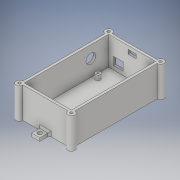
# Autodesk Inventor part: Podstawa
Saved by Autodesk Inventor 2019 (Build 230136000, 136)
## iProperties
Created: 2019-09-16
Part Number: Podstawa
Material: Ogólny
Document SubType Name: Modeling
Designer: mikol
Density: 1 g/cm^3
Appearance: Domyślna
Author: mikol
Autodesk Inventor part; units mm, degrees
ref_plane "YZ Plane" through (0, 0, 0) normal (1, 0, 0) x (0, 1, 0)
ref_plane "XZ Plane" through (0, 0, 0) normal (0, 1, 0) x (-1, 0, 0)
ref_plane "XY Plane" through (0, 0, 0) normal (0, 0, 1) x (1, 0, 0)
sketch "Sketch1" plane through (0, 0, 0) normal (0, 1, 0) x (-1, 0, 0)
  line L0 (32, 55) -> (-32, 55)
  line L1 (-32, 55) -> (-32, -55)
  line L2 (-32, -55) -> (32, -55)
  line L3 (32, -55) -> (32, 55)
  line L4 (32, 55) -> (-32, -55) construction
  line L5 (-32, 55) -> (32, -55) construction
  point P0 (0, 0)
  dimension "d0" = 64
  dimension "d1" = 110
  constraints: 12 end point, 2 midpoint, 2 parallel, 1 horizontal, 1 perpendicular
  measures "d0" distance of L2.end L1.end
  measures "d1" distance of L1.end L0.end
extrude "Extrusion1" add sketch "Sketch1" along normal blind 3
sketch "Sketch2" plane through (0, 3, 0) normal (0, 1, 0) x (1, 0, 0)
  line L0 (-32, -55) -> (32, -55) projected
  line L1 (32, -55) -> (32, 55) projected
  line L2 (32, 55) -> (-32, 55) projected
  line L3 (-32, 55) -> (-32, -55) projected
  line L4 (-32, -55) -> (32, -55)
  line L5 (32, -55) -> (32, 55)
  line L6 (32, 55) -> (-32, 55)
  line L7 (-32, 55) -> (-32, -55)
  line L8 (-32, -55) -> (32, 55) construction
  line L9 (32, -55) -> (-32, 55) construction
  line L10 (-29, -52) -> (29, -52)
  line L11 (29, -52) -> (29, 52)
  line L12 (29, 52) -> (-29, 52)
  line L13 (-29, 52) -> (-29, -52)
  point P0 (0, 0)
  dimension "d4" = 3
  dimension "d5" = 3
  dimension "d6" = 3
  dimension "d7" = 3
  constraints: 20 end point, 4 parallel, 2 horizontal, 2 midpoint, 2 perpendicular
  measures "d4" distance between parallel lines of L2 L12
  measures "d5" distance between parallel lines of L7 L13
  measures "d6" distance between parallel lines of L0 L10
  measures "d7" distance between parallel lines of L1 L11
extrude "Extrusion2" add sketch "Sketch2" along normal blind 35
sketch "Sketch3" plane through (0, 3, 0) normal (0, 1, 0) x (1, 0, 0)
  line L0 (-23.08, -46) -> (23.08, -46)
  line L1 (23.08, -46) -> (23.08, 46)
  line L2 (23.08, 46) -> (-23.08, 46)
  line L3 (-23.08, 46) -> (-23.08, -46)
  circle A0 centre (-23.08, -46) radius 1.25
  circle A1 centre (23.08, -46) radius 1.25
  circle A2 centre (23.08, 46) radius 1.25
  circle A3 centre (-23.08, 33) radius 1.25
  line L4 (-29, -52) -> (-29, 52) projected
  line L5 (29, 52) -> (29, -52) projected
  line L6 (-29, 52) -> (29, 52) projected
  line L7 (29, -52) -> (-29, -52) projected
  circle A4 centre (-23.08, -46) radius 3
  circle A5 centre (-23.08, 33) radius 3
  circle A6 centre (23.08, -46) radius 3
  circle A7 centre (23.08, 46) radius 3
  point P0 (0, 0)
  dimension "d15" = 46.16
  dimension "d16" = 92
  dimension "d17" = 2.5
  dimension "d18" = 2.5
  dimension "d19" = 2.5
  dimension "d20" = 2.5
  dimension "d21" = 79
  dimension "d22" = 5.92
  dimension "d23" = 5.92
  dimension "d24" = 6
  dimension "d25" = 6
  dimension "d26" = 6
  dimension "d27" = 6
  dimension "d28" = 6
  dimension "d29" = 6
  constraints: 8 centre point, 8 end point, 7 coincident, 2 parallel, 1 horizontal, 1 perpendicular, 1 point on line
  measures "d15" distance of L2.end L1.end
  measures "d16" distance of L1.end L0.end
  measures "d17" diameter of A0
  measures "d18" diameter of A1
  measures "d19" diameter of A2
  measures "d20" diameter of A3
  measures "d21" distance of A3.centre L0.start
  measures "d22" distance between parallel lines of L4 L3
  measures "d23" distance between parallel lines of L5 L1
  measures "d24" distance between parallel lines of L6 L2
  measures "d25" distance between parallel lines of L7 L0
  measures "d26" diameter of A4
  measures "d27" diameter of A5
  measures "d28" diameter of A6
  measures "d29" diameter of A7
extrude "Extrusion3" add sketch "Sketch3" along normal blind 6 contours A0 L3 A4 L0 | L0 A4 L3 A0 | A6 L1 A1 L0 | L0 A1 L1 A6 | A5 L3 A3 | L3 A3 A5 | A7 L2 A2 L1 | L1 A2 L2 A7
sketch "Sketch4" plane through (-29, 3, -52) normal (0, 0, 1) x (1, 0, 0)
  line L0 (8.92, 6) -> (2.92, 6) projected
  line L1 (5.92, 4.5) -> (17.92, 4.5)
  line L2 (17.92, 4.5) -> (17.92, 14.5)
  line L3 (17.92, 14.5) -> (5.92, 14.5)
  line L4 (5.92, 14.5) -> (5.92, 4.5)
  point P0 (29, -3)
  dimension "d33" = 1.5
  dimension "d34" = 10
  dimension "d35" = 12
  constraints: 8 end point, 2 parallel, 1 horizontal, 1 perpendicular
  measures "d33" distance between parallel lines of L0 L1
  measures "d34" distance between parallel lines of L3 L1
  measures "d35" distance between parallel lines of L2 L4
extrude "Extrusion4" cut sketch "Sketch4" against normal blind 6
sketch "Sketch5" plane through (-29, 3, -52) normal (0, 0, 1) x (1, 0, 0)
  line L0 (17.92, 14.5) -> (17.92, 4.5) projected
  line L1 (17.92, 4.5) -> (5.92, 4.5) projected
  line L2 (5.92, 4.5) -> (5.92, 14.5) projected
  line L3 (5.92, 14.5) -> (17.92, 14.5) projected
  line L4 (58, 0) -> (0, 0) projected
  line L5 (58, 0) -> (58, 35) projected
  line L6 (0, 35) -> (58, 35) projected
  line L7 (0, 0) -> (0, 35) projected
  line L8 (24, 31) -> (34, 31)
  line L9 (34, 31) -> (34, 26)
  line L10 (34, 26) -> (24, 26)
  line L11 (24, 26) -> (24, 31)
  line L12 (8.92, 6) -> (2.92, 6) projected
  point P0 (29, -3)
  dimension "d38" = 20
  dimension "d39" = 5
  dimension "d40" = 10
  dimension "d41" = 24
  dimension "d42" = 24
  constraints: 8 end point, 2 parallel, 1 horizontal, 1 perpendicular
  measures "d38" distance between parallel lines of L10 L12
  measures "d39" distance between parallel lines of L10 L8
  measures "d40" distance between parallel lines of L9 L11
  measures "d41" distance between parallel lines of L7 L11
  measures "d42" distance between parallel lines of L5 L9
extrude "Extrusion5" cut sketch "Sketch5" against normal blind 6 contours L8 L9 L10 L11
sketch "Sketch7" plane through (0, 0, 0) normal (0, -1, 0) x (1, 0, 0)
  line L0 (29, 52) -> (-29, 52) projected
  line L1 (-29, 52) -> (-29, -52) projected
  line L2 (-29, -52) -> (29, -52) projected
  line L3 (29, -52) -> (29, 52) projected
  line L4 (29, 52) -> (-29, 52) projected
  line L5 (32, -55) -> (-32, -55) projected
  line L6 (-32, -55) -> (-32, 55) projected
  line L7 (-32, 55) -> (32, 55) projected
  line L8 (32, 55) -> (32, -55) projected
  line L9 (32, 55) -> (32, -55) projected
  circle A0 centre (32, 55) radius 4.2426
  point P0 (0, 0)
  constraints: 1 coincident, 3 other
extrude "Extrusion6" add sketch "Sketch7" against normal blind 38 contours A0 L7 L8 | A0 L8 L7
sketch "Sketch8" plane through (0, 38, 0) normal (0, 1, 0) x (1, 0, 0)
  arc A0 (27.7574, -55) -> (32, -50.7574) centre (32, -55) ccw projected
  circle A1 centre (32, -55) radius 1.65
  point P0 (0, 0)
  dimension "d47" = 3.3
  constraints: 1 centre point, 1 coincident
  measures "d47" diameter of A1
extrude "Extrusion7" cut sketch "Sketch8" against normal blind 15
mirror "Mirror1" about plane through (0, 0, 0) normal (1, 0, 0) of "Extrusion6", "Extrusion7"
mirror "Mirror2" about plane through (0, 0, 0) normal (0, 0, 1) of "Extrusion6", "Extrusion7", "Mirror1"
sketch "Sketch9" plane through (-29, 3, 52) normal (1, 0, 0) x (0, 0, -1)
  line L0 (88, 6) -> (82, 6) projected
  circle A0 centre (82, 20) radius 6
  line L1 (85, 6) -> (85, 35)
  line L2 (0, 35) -> (104, 35) projected
  line L3 (85, 6) -> (114, 6) construction
  point P0 (52, -3)
  dimension "d50" = 12
  dimension "d51" = 14
  dimension "d52" = 90
  dimension "d53" = 3
  constraints: 4 end point, 1 centre point, 1 horizontal, 1 midpoint, 1 perpendicular, 1 point on line
  measures "d50" diameter of A0
  measures "d51" distance from line of A0.centre L0
  measures "d52" angle of L3 L1
  measures "d53" distance from line of L1 A0.centre
extrude "Extrusion8" cut sketch "Sketch9" against normal through all
sketch "Sketch10" plane through (27.7574, 0, -55) normal (0, 0, -1) x (-1, 0, 0)
  line L0 (22.7574, 0) -> (32.7574, 0)
  line L1 (32.7574, 0) -> (32.7574, 4)
  line L2 (32.7574, 4) -> (22.7574, 4)
  line L3 (22.7574, 4) -> (22.7574, 0)
  line L4 (55.5147, 0) -> (55.5147, 38) projected
  line L5 (0, 38) -> (0, 0) projected
  point P0 (27.7574, 0)
  dimension "d56" = 4
  dimension "d57" = 10
  dimension "d58" = 22.7574
  dimension "d59" = 22.7574
  constraints: 8 end point, 2 parallel, 1 horizontal, 1 perpendicular
  measures "d56" distance of L0.end L1.end
  measures "d57" distance of L1.end L2.end
  measures "d58" distance between parallel lines of L4 L1
  measures "d59" distance between parallel lines of L5 L3
extrude "Extrusion9" add sketch "Sketch10" along normal blind 12
chamfer "Chamfer1" distance 2 angle 45 3 edges at (5, 2, -55) (-5, 2, -55) (0, 4, -55)
sketch "Sketch11" plane through (-5, 4, -67) normal (0, 1, 0) x (1, 0, 0)
  line L0 (10, -10) -> (0, -10) projected
  line L1 (10, -10) -> (10, 0) projected
  line L2 (0, 0) -> (10, 0) projected
  line L3 (0, -10) -> (0, 0) projected
  circle A0 centre (5, -5) radius 2.6
  point P0 (5, -67)
  dimension "d65" = 5.2
  dimension "d66" = 5
  dimension "d67" = 5
  constraints: 1 centre point
  measures "d65" diameter of A0
  measures "d66" distance from line of L3 A0.centre
  measures "d67" distance from line of L2 A0.centre
extrude "Extrusion10" cut sketch "Sketch11" against normal through all contours A0
mirror "Mirror3" about plane through (0, 0, 0) normal (0, 0, 1) of "Extrusion9", "Extrusion10"
chamfer "Chamfer2" distance 2 angle 45 3 edges at (-5, 2, 55) (0, 4, 55) (5, 2, 55)
equation "\"d4\" = d5"
equation "\"d6\" = d5"
equation "\"d7\" = d5"
equation "\"d22\" = d23"
equation "\"d24\" = d25"
equation "\"d27\" = d26"
equation "\"d28\" = d26"
equation "\"d29\" = d26"
equation "\"d41\" = d42"
equation "\"d58\" = d59"
body "Solid1"
